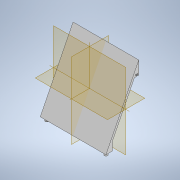
# Autodesk Inventor part: Roof_Large
Saved by Autodesk Inventor 2022.4 (Build 264492010, 492A)
## iProperties
Created: 2025-02-20
Part Number: Roof_Large
Material: Generic
Document SubType Name: Modeling
Designer: jan-m
Density: 1 g/cm^3
Appearance: Default
Author: jan-m
Autodesk Inventor part; units mm, degrees
sketch "Sketch1" plane through (0, 0, 0) normal (1, 0, 0) x (0, 1, 0)
  line L0 (50, 25) -> (-50, 25)
  line L1 (-50, 25) -> (-50, -25)
  line L2 (-50, -25) -> (50, -25)
  line L3 (50, -25) -> (50, 25)
  line L4 (-70, 0) -> (70, 0) projected
  line L5 (0, 35) -> (0, -35) projected
  line L6 (-50, 25) -> (50, -25)
  line L7 (-36.7082, 15) -> (30, -18.3541)
  line L8 (-36.7082, 15) -> (-50, 15)
  line L9 (30, -25) -> (30, -18.3541)
  line L10 (30, -21.8) -> (33, -21.8)
  line L11 (33, -21.8) -> (33, -23.4)
  line L12 (33, -23.4) -> (30, -23.4)
  line L13 (30, -23.4) -> (30, -21.8)
  line L14 (33, -21.8) -> (31.4, -21.8)
  line L15 (31.4, -21.8) -> (31.4, -20.2)
  line L16 (31.4, -20.2) -> (33, -20.2)
  line L17 (33, -20.2) -> (33, -21.8)
  point P0 (0, 0)
  point P1 (50, 0)
  point P2 (0, 25)
  point P3 (43.2918, -25)
  point P4 (-50, 21.6459)
  dimension "d0" = 50
  dimension "d1" = 100
  dimension "d2" = 3
  dimension "d5" = 10
  dimension "d6" = 20
  dimension "d95" = 3
  dimension "d96" = 1.6
  dimension "d97" = 1.6
  dimension "d98" = 1.6
  dimension "d99" = 1.6
  constraints: 34 end point, 7 parallel, 5 point on line, 4 perpendicular, 3 horizontal, 2 midpoint, 1 vertical
  measures "d0" distance of L2.end L0.start
  measures "d1" distance of L1.end L2.end
  measures "d2" distance between parallel lines of L6 L7
  measures "d5" distance between parallel lines of L0 L8
  measures "d6" distance between parallel lines of L3 L9
  measures "d95" distance of L11.end L12.end
  measures "d96" distance of L10.end L11.end
  measures "d97" distance between parallel lines of L2 L12
  measures "d98" distance of L15.end L16.end
  measures "d99" distance of L16.end L10.end
extrude "Extrusion1" add sketch "Sketch1" along normal mid plane 100 contours L6 L4 L7 L8 L1 | L5 L7 L4 | L6 L2 L9 L12 L11 L17 L16 L15 L10 L7 L5
sketch "Sketch4" plane through (50, 50, -25) normal (0, 0, -1) x (-1, 0, 0)
  circle A0 centre (5, -5) radius 1.5
  line L0 (0, -20) -> (0, 0) projected
  line L1 (100, 0) -> (0, 0) projected
  line L2 (5, -3.5) -> (5, -6.5)
  circle A1 centre (35, -5) radius 1.5
  line L3 (35, -3.5) -> (35, -6.5)
  circle A2 centre (65, -5) radius 1.5
  line L4 (65, -3.5) -> (65, -6.5)
  circle A3 centre (95, -5) radius 1.5
  line L5 (95, -3.5) -> (95, -6.5)
  point P0 (50, -50)
  point P1 (0, -100)
  dimension "d45" = 3
  dimension "d46" = 5
  dimension "d47" = 5
  dimension "d48" = 3
  dimension "d107" = 3
  dimension "d108" = 5
  dimension "d109" = 30
  dimension "d110" = 3
  dimension "d120" = 60
  dimension "d127" = 60
  constraints: 8 end point, 8 point on circle, 4 centre point, 2 horizontal, 2 vertical, 1 midpoint, 11 other
  measures "d45" diameter of A0
  measures "d46" distance from line of L0 A0.centre
  measures "d47" distance from line of L1 A0.centre
  measures "d48" distance of L2.start L2.end
  measures "d107" diameter of A1
  measures "d108" distance from line of L1 A1.centre
  measures "d109" distance of point (5, -5) A1.centre
  measures "d110" distance of L3.start L3.end
  measures "d120" distance of A0.centre A2.centre
  measures "d127" distance of A1.centre A3.centre
revolve "Revolution2" add sketch "Sketch4" angle 360 about axis through (45, 46.5, -25) along (0, -1, 0) picked at (4.5036, -4.9397) contours L2 A0
revolve "Revolution3" cut sketch "Sketch4" angle 360 about axis through (15, 46.5, -25) along (0, -1, 0) picked at (34.5036, -5.0603) contours L3 A1
revolve "Revolution4" add sketch "Sketch4" angle 360 about axis through (-15, 46.5, -25) along (0, -1, 0) picked at (64.2365, -5.2413) contours L4 A2
revolve "Revolution5" cut sketch "Sketch4" angle 360 about axis through (-45, 46.5, -25) along (0, -1, 0) picked at (94.1238, -4.716) contours L5 A3
sketch "Sketch5" plane through (-50, -50, 15) normal (0, -1, 0) x (1, 0, 0)
  circle A0 centre (5, 5) radius 2.5
  line L0 (0, 0) -> (0, 10) projected
  line L1 (0, 10) -> (100, 10) projected
  line L2 (50, 20) -> (50, -50) projected
  circle A1 centre (95, 5) radius 2.5
  line L3 (0, 5) -> (100, 5)
  line L4 (100, -40) -> (100, 10) projected
  point P0 (50, -15)
  dimension "d76" = 5
  dimension "d77" = 5
  constraints: 2 centre point, 2 end point, 2 point on line, 1 horizontal, 1 midpoint, 1 symmetric about line, 1 other
  measures "d76" diameter of A0
  measures "d77" distance from line of L0 A0.centre
extrude "Extrusion3" add sketch "Sketch5" along normal blind 5 contours L3 A0 | A0 L3 | L3 A1 | A1 L3
body "Solid1"
